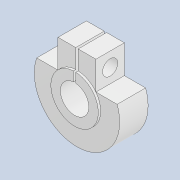
# Autodesk Inventor part: shooter_base7
Saved by Autodesk Inventor 2022 (Build 260153000, 153)
## iProperties
Created: 2021-05-27
Part Number: shooter_base7
Material: ABS プラスチック
Document SubType Name: Modeling
Designer: yuta0
Density: 1.06 g/cm^3
Appearance: 滑らか - 白
Author: yuta0
Autodesk Inventor part; units mm, degrees
ref_plane "XZ Plane" through (0, 0, 0) normal (0, 1, 0) x (-1, 0, 0)
ref_plane "XY Plane" through (0, 0, 0) normal (0, 0, 1) x (1, 0, 0)
sketch "スケッチ1" plane through (0, 0, 0) normal (0, 0, 1) x (1, 0, 0)
  circle A0 centre (0, 0) radius 3
  circle A1 centre (0, 0) radius 9
  dimension "d0" = 6
  dimension "d1" = 18
  constraints: 2 centre point, 2 coincident
  measures "d0" diameter of A0
  measures "d1" diameter of A1
extrude "押し出し1" add sketch "スケッチ1" along normal mid plane 6
ref_plane "作業平面1" through (-9, 0, 0) normal (1, 0, 0) x (0, 1, 0)
sketch "スケッチ5" plane through (0, 0, 3) normal (0, 0, 1) x (1, 0, 0)
  arc A0 (3, 0) -> (3, 0) centre (0, 0) ccw projected
  circle A1 centre (0, 0) radius 5
  circle A2 centre (0, 0) radius 3 projected
  circle A3 centre (0, 0) radius 3 projected
  dimension "d33" = 10
  constraints: 1 centre point, 1 coincident
  measures "d33" diameter of A1
extrude "押し出し3" add sketch "スケッチ5" along normal blind 0.5
chamfer "面取り3" distance 0.5 angle 45 1 edges at (-3, 0, -3)
sketch "スケッチ10" plane through (0, 0, -3) normal (0, 0, -1) x (-1, 0, 0)
  circle A0 centre (0, 0) radius 9 projected
  line L0 (-9, 9) -> (-4, 9)
  line L1 (-4, 9) -> (-4, 3)
  line L2 (-4, 3) -> (-9, 3)
  line L3 (-9, 3) -> (-9, 9)
  point P0 (-8.4853, 3)
  point P1 (-4, 8.0623)
  dimension "d48" = 4
  dimension "d49" = 6
  constraints: 8 end point, 2 parallel, 2 tangent, 1 horizontal, 1 perpendicular
  measures "d48" distance from line of point (0, 0) L1
  measures "d49" distance of L0.end L1.end
extrude "押し出し7" cut sketch "スケッチ10" against normal blind 10 contours L1 L2 A0 picked at (-4.4898, 6.0699)
mirror "ミラー4" about plane through (0, 0, 0) normal (1, 0, 0) of "押し出し7"
sketch "スケッチ11" plane through (-4, 3, 3) normal (-1, 0, 0) x (0, 0, 1)
  line L0 (-7.3, -3) -> (1.8, -3) projected
  line L1 (-6, 0) -> (-6, 5.0623) projected
  point P0 (-3, -3)
  point P1 (-3, 3)
  dimension "d52" = 6
  dimension "d53" = 3
  measures "d52" distance from line of point (-3, 3) L0
  measures "d53" distance from line of L1 point (-3, 3)
hole "穴3" at (-4, 6, 0) direction (1, 0, 0) diameter 3.2 end through all clearance for "Socket Head Cap Screw" size "M3" standard "Ansi Metric M Profile"
sketch "スケッチ12" plane through (0, 0, -3) normal (0, 0, -1) x (-1, 0, 0)
  line L0 (-4, 8.0623) -> (4, 8.0623)
  line L1 (4, 8.0623) -> (4, 9)
  line L2 (4, 9) -> (-4, 9)
  line L3 (-4, 9) -> (-4, 8.0623)
  arc A0 (4, 8.0623) -> (-4, 8.0623) centre (0, 0) ccw projected
  point P0 (0, 9)
  constraints: 8 end point, 2 parallel, 1 horizontal, 1 perpendicular, 1 tangent
extrude "押し出し8" add sketch "スケッチ12" against normal up to surface (6 mm away) contours L3 L2 A0 | A0 L2 L1
sketch "スケッチ13" plane through (0, 0, -3) normal (0, 0, -1) x (-1, 0, 0)
  line L0 (-0.25, 9) -> (0.25, 9)
  line L1 (0.25, 9) -> (0.25, 2.9896)
  line L2 (0.25, 2.9896) -> (-0.25, 2.9896)
  line L3 (-0.25, 2.9896) -> (-0.25, 9)
  line L4 (-0.25, 9) -> (0.25, 2.9896) construction
  line L5 (0.25, 9) -> (-0.25, 2.9896) construction
  line L6 (4, 9) -> (-4, 9) projected
  circle A0 centre (0, 0) radius 3 projected
  point P0 (0, 5.9948)
  point P1 (0, 5.9948)
  dimension "d63" = 0.5
  constraints: 12 end point, 3 midpoint, 2 parallel, 1 horizontal, 1 perpendicular, 1 point on line, 1 vertical alignment, 2 other
  measures "d63" distance of L0.start L0.end
extrude "押し出し9" cut sketch "スケッチ13" against normal blind 10 contours L0 L1 A0 L3
